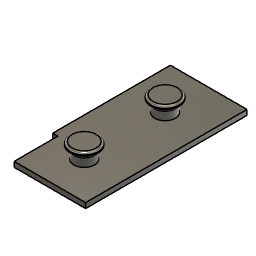
PCB+STM_LID v7 (Autodesk Fusion 360 design; units mm, degrees)
Autodesk Fusion 360 part; units mm, degrees
sketch "Sketch1" plane through (0, 0, 0) normal (0, 1, 0) x (1, 0, 0)
  line L0 (0, 0) -> (74.5, 0)
  line L1 (74.5, 0) -> (74.5, -114.4)
  line L2 (74.5, -114.4) -> (0, -114.4)
  line L3 (0, -114.4) -> (0, 0)
  dimension "d1" = 74.5
  dimension "d2" = 114.4
  constraint horizontal L0
  constraint vertical L1
  constraint horizontal L2
  constraint vertical L3
  constraint coincident L0.start L3.end
  measures "d1" distance of L0.start L0.end
  measures "d2" distance of L0.start L2.end
extrude "Extrude1" add sketch "Sketch1" along normal blind 5
sketch "Sketch2" plane through (0, 5, 0) normal (0, 1, 0) x (-1, 0, 0)
  line L0 (0, 114.4) -> (-74.5, 114.4)
  line L1 (-74.5, 114.4) -> (-74.5, 0)
  line L2 (-74.5, 0) -> (0, 0)
  line L3 (0, 0) -> (0, 114.4)
  line L4 (0, 114.4) -> (-5, 114.4)
  line L5 (-5, 114.4) -> (-74.5, 114.4)
  line L6 (-74.5, 114.4) -> (-74.5, 157)
  line L7 (-74.5, 157) -> (-5, 157)
  line L8 (-5, 157) -> (-5, 114.4)
  dimension "d5" = 5
  dimension "d6" = 69.5
  dimension "d7" = 42.6
  constraint coincident L0.start L3.end
  constraint perpendicular L3 L4
  constraint horizontal L5
  constraint vertical L6
  constraint horizontal L7
  constraint vertical L8
  measures "d5" distance of L0.start L4.end
  measures "d6" distance of L4.end L0.end
  measures "d7" distance of L4.end L7.end
extrude "Extrude2" add sketch "Sketch2" against normal blind 5 contours L0 L5 L6 L7 L8
sketch "Sketch5" plane through (0, 5, 0) normal (0, 1, 0) x (-1, 0, 0)
  line L0 (0, 114.4) -> (-5, 114.4)
  line L1 (-5, 114.4) -> (-5, 157)
  line L2 (-5, 157) -> (-74.5, 157)
  line L3 (-74.5, 157) -> (-74.5, 0)
  line L4 (-74.5, 0) -> (0, 0)
  line L5 (0, 0) -> (0, 114.4)
  circle A0 centre (-37.1142, 42.2817) radius 10
  dimension "d21" = 20
  measures "d21" diameter of A0
extrude "Extrude3" add sketch "Sketch5" along normal blind 10 contours A0
sketch "Sketch6" plane through (0, 15, 0) normal (0, 1, 0) x (-1, 0, 0)
  circle A0 centre (-37.1142, 42.2817) radius 10
  circle A1 centre (-37.1142, 42.2817) radius 13.7352
  constraint concentric A0 A1
extrude "Extrude4" add sketch "Sketch6" along normal blind 5 contours A0 | A1
fillet "Fillet1" radius 2 1 edges at (46.4375, 15, 38.6655)
fillet "Fillet2" radius 2 2 edges at (49.9199, 15, 37.3148) (49.9199, 20, 37.3148)
sketch "Sketch7" plane through (0, 5, 0) normal (0, 1, 0) x (-1, 0, 0)
  circle A0 centre (-37.1142, 42.2817) radius 10
  line L0 (0, 114.4) -> (-5, 114.4)
  line L1 (-5, 114.4) -> (-5, 157)
  line L2 (-5, 157) -> (-74.5, 157)
  line L3 (-74.5, 157) -> (-74.5, 0)
  line L4 (-74.5, 0) -> (0, 0)
  line L5 (0, 0) -> (0, 114.4)
  circle A1 centre (-37.1142, 120.9425) radius 10
  dimension "d30" = 20
  measures "d30" diameter of A1
extrude "Extrude5" add sketch "Sketch7" along normal blind 10 contours A1
sketch "Sketch8" plane through (0, 15, 0) normal (0, 1, 0) x (-1, 0, 0)
  circle A0 centre (-37.1142, 120.9425) radius 10
  circle A1 centre (-37.1142, 120.9425) radius 13.6136
  constraint concentric A0 A1
extrude "Extrude6" add sketch "Sketch8" along normal blind 5 contours A0 | A1
fillet "Fillet3" radius 2 1 edges at (46.4375, 15, 117.3263)
fillet "Fillet4" radius 2 2 edges at (49.8066, 15, 116.0196) (49.8066, 20, 116.0196)
